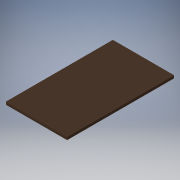
# Autodesk Inventor part: adapter
Saved by Autodesk Inventor 2019 (Build 230136000, 136)
## iProperties
Created: 2019-04-29
Part Number: adapter
Material: Bronze, Soft Tin
Document SubType Name: Modeling
Designer: Alex
Density: 8.874 g/cm^3
Appearance: Bronze - Satin
Author: Alex
Autodesk Inventor part; units mm, degrees
ref_plane "YZ Plane" through (0, 0, 0) normal (1, 0, 0) x (0, 1, 0)
ref_plane "XZ Plane" through (0, 0, 0) normal (0, 1, 0) x (-1, 0, 0)
ref_plane "XY Plane" through (0, 0, 0) normal (0, 0, 1) x (1, 0, 0)
sketch "Sketch1" plane through (0, 0, 0) normal (0, 1, 0) x (-1, 0, 0)
  line L0 (196.6697, 476.1405) -> (-403.3303, 476.1405)
  line L1 (-403.3303, 476.1405) -> (-403.3303, -573.8595)
  line L2 (-403.3303, -573.8595) -> (196.6697, -573.8595)
  line L3 (196.6697, -573.8595) -> (196.6697, 476.1405)
  point P0 (0, 0)
  dimension "d0" = 1050
  dimension "d1" = 600
  constraints: 8 end point, 2 parallel, 1 horizontal, 1 perpendicular
  measures "d0" distance between parallel lines of L2 L0
  measures "d1" distance between parallel lines of L1 L3
extrude "Extrusion1" add sketch "Sketch1" along normal blind 27
body "Solid1"
